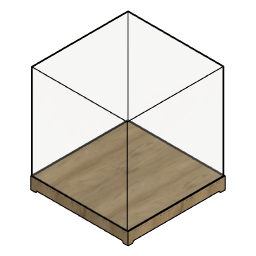
Base_paraiso (Autodesk Fusion 360 design; units mm, degrees)
Autodesk Fusion 360 part; units mm, degrees
sketch "Sketch3" plane through (0, 0, 0) normal (0, 0, 1) x (1, 0, 0)
  line L0 (-400, -400) -> (400, -400)
  line L1 (400, -400) -> (400, 400)
  line L2 (400, 400) -> (-400, 400)
  line L3 (-400, 400) -> (-400, -400)
  line L4 (382, -382) -> (382, 382)
  line L5 (382, 382) -> (-382, 382)
  line L6 (-382, 382) -> (-382, -382)
  line L7 (-382, -382) -> (382, -382)
  line L8 (-400, 400) -> (-382, 382)
  line L9 (382, -382) -> (400, -400)
  line L10 (-400, -400) -> (-382, -382)
  line L11 (382, 382) -> (400, 400)
  line L12 (-400, -400) -> (-382, -382) construction
  line L13 (382, 382) -> (400, 400) construction
  line L14 (400, -400) -> (382, -382) construction
  line L15 (-382, 382) -> (-400, 400) construction
  dimension "d11" = 800
  dimension "d12" = 800
  dimension "d13" = -18
  constraint horizontal L0
  constraint perpendicular L0 L1
  constraint parallel L0 L2
  constraint parallel L1 L3
  constraint coincident origin L12
  constraint coincident origin L14
  constraint parallel L8 L14
  constraint collinear L8 L9
  constraint collinear L10 L11
  constraint collinear L12 L13
  constraint collinear L14 L15
  measures "d11" distance of L1.end L2.end
  measures "d12" distance of L0.end L1.end
extrude "Extrude3" add sketch "Sketch3" along normal blind 100 contours L3 L6 L8 L10 | L1 L4 L9 L11 makes body 1 at (-400, 133.3333, 66.6667) makes body 2 at (400, -133.3333, 66.6667)
extrude "Extrude4" add sketch "Sketch3" along normal blind 100 separate body contours L0 L7 L9 L10 | L2 L5 L8 L11 makes body 3 at (-133.3333, -400, 66.6667) makes body 4 at (133.3333, 400, 66.6667)
sketch "Sketch4" plane through (0, -400, 0) normal (0, -1, 0) x (1, 0, 0)
  line L0 (-400, 0) -> (400, 0)
  line L1 (400, 0) -> (400, 100)
  line L2 (400, 100) -> (-400, 100)
  line L3 (-400, 100) -> (-400, 0)
  line L4 (-350, 0) -> (0, 0)
  line L5 (-350, 15) -> (0, 15)
  line L6 (-350, 0) -> (-365, 0)
  arc A0 (-350, 15) -> (-365, 0) centre (-350, 0) ccw
  spline S0 degree 5 poles (0, 0) (0, 7.6752) (0, 23.0256) (0, 46.0513) (0, 76.7521) (0, 115.1282) (0, 145.829) (0, 168.8546) (0, 184.2051) (0, 191.8803) knots 0 0 0 0 0 0 0.2 0.4 0.6 0.8 1 1 1 1 1 1 construction
  line L7 (0, 1.75) -> (0, 22.5) construction
  line L8 (350, 0) -> (0, 0)
  line L9 (350, 0) -> (365, 0)
  arc A1 (365, 0) -> (350, 15) centre (350, 0) ccw
  line L10 (350, 15) -> (0, 15)
  point P0 (-400, 0)
  dimension "d18" = -15
  dimension "d19" = 50
  constraint coincident L0 L4.start
  constraint coincident L4.end S0.start
  constraint perpendicular L3 L4
  constraint coincident L4.start L6.start
  constraint tangent L5 A0
  constraint coincident L0 L6.end
  constraint symmetric L4.start L7 L8.start
  constraint symmetric L4.end L7 S0.start
  constraint symmetric L5.start L7 A1.end
  constraint symmetric L5.end L7 L10.end
  constraint symmetric L6.end L7 L9.end
  constraint symmetric A0 L7 A1
  measures "d19" distance of L4.start P0
ref_plane "WorkPlane1" through (0, -400, 50) normal (0, -1, 0) x (1, 0, 0)
sketch "Sketch6" plane through (0, 0, 100) normal (0, 0, 1) x (-1, 0, 0)
  line L0 (400, 400) -> (-400, 400)
  line L1 (-400, 400) -> (-382, 382)
  line L2 (-382, 382) -> (382, 382)
  line L3 (382, 382) -> (400, 400)
  line L4 (394, 394) -> (-394, 394)
  line L5 (-394, 394) -> (-394, -394)
  line L6 (-394, -394) -> (394, -394)
  line L7 (394, -394) -> (394, 394)
  line L8 (394, 394) -> (-394, -394) construction
  line L9 (-394, 394) -> (394, -394) construction
  dimension "d38" = 12
  constraint horizontal L4
  constraint perpendicular L4 L5
  constraint parallel L4 L6
  constraint parallel L5 L7
  constraint coincident L8 origin
  constraint coincident L9 origin
  measures "d38" distance of L2 L4
extrude "Extrude8" cut sketch "Sketch6" against normal blind 20 contours L1 L2 L3 L5 L6 L7 | L1 L2 L3 L4 bodies 1 2 3 4
sketch "Sketch11" plane through (0, -400, 0) normal (0, -1, 0) x (1, 0, 0)
  line L0 (0, 0) -> (0, 171.862) construction
  line L1 (-360, 0) -> (-360, -0.0001)
  line L2 (-345, 15) -> (0, 15)
  arc A0 (-345, 15) -> (-360, -0.0001) centre (-345, 0) ccw
  line L3 (-360, 0) -> (0, 0)
  line L4 (345, 15) -> (0, 15)
  line L5 (360, 0) -> (0, 0)
  arc A1 (360, -0.0001) -> (345, 15) centre (345, 0) ccw
  point P0 (-360.0001, 15)
  point P1 (-400, 0)
  dimension "d67" = 15
  dimension "d68" = 40
  dimension "d69" = 15
  constraint coincident L0.start L3.end
  constraint vertical L0
  constraint coincident L0 L2.end
  constraint perpendicular L0 L2
  constraint coincident P0 L1
  constraint coincident P0 L2
  constraint tangent L1 A0
  constraint tangent L2 A0
  constraint perpendicular L0 L3
  constraint symmetric L0 L1.start L5.start
  constraint symmetric L0 L2.end L4.end
  constraint symmetric L0 L1.end A1.start
  constraint symmetric L0 L2.start L4.start
  constraint symmetric L0 A0 A1
  constraint symmetric L0 L3.end L5.end
  measures "d67" distance of L1.start P0
  measures "d68" distance of L1.start P1
  measures "d69" radius of A0
extrude "Extrude12" cut sketch "Sketch11" against normal blind 840 bodies 3 4
sketch "Sketch12" plane through (-400, 0, 0) normal (-1, 0, 0) x (0, -1, 0)
  line L0 (-400, 0) -> (400, 0)
  line L1 (400, 0) -> (400, 100)
  line L2 (400, 100) -> (-400, 100)
  line L3 (-400, 100) -> (-400, 0)
  line L4 (0, 0) -> (0, 212.8854) construction
  line L5 (-360, 0) -> (-360, 0.5)
  line L6 (-345.5, 15) -> (0, 15)
  arc A0 (-345.5, 15) -> (-360, 0.5) centre (-345.5, 0.5) ccw
  line L7 (-360, 0) -> (0, 0)
  line L8 (345.5, 15) -> (0, 15)
  arc A1 (360, 0.5) -> (345.5, 15) centre (345.5, 0.5) ccw
  line L9 (360, 0) -> (0, 0)
  line L10 (360, 0.5) -> (360, 0)
  point P0 (-360, 15)
  dimension "d76" = 40
  dimension "d77" = 15
  dimension "d78" = 14.5
  constraint coincident L4.start L7.end
  constraint perpendicular L0 L4
  constraint coincident L0 L5.start
  constraint perpendicular L0 L5
  constraint coincident L4 L6.end
  constraint perpendicular L4 L6
  constraint coincident P0 L5
  constraint coincident P0 L6
  constraint tangent L5 A0
  constraint tangent L6 A0
  constraint symmetric L4 L5.start L9.start
  constraint symmetric L4 L6.end L8.end
  constraint symmetric L4 L5.end A1.start
  constraint symmetric L4 L6.start L8.start
  constraint symmetric L4 A0 A1
  constraint symmetric L4 L7.end L9.end
  measures "d76" distance of L0.start L5.start
  measures "d77" distance of L5.start P0
  measures "d78" radius of A0
extrude "Extrude13" cut sketch "Sketch12" against normal blind 950 contours L0 L5 L6 A0 L7 L8 A1 L9 L10 bodies 2 1
sketch "Sketch13" plane through (0, 0, 100) normal (0, 0, 1) x (-1, 0, 0)
  line L0 (394, -394) -> (-394, -394)
  line L1 (-394, -394) -> (-400, -400)
  line L2 (-400, -400) -> (400, -400)
  line L3 (400, -400) -> (394, -394)
  line L4 (391, -391) -> (-391, -391)
  line L5 (-391, -391) -> (-391, 391)
  line L6 (-391, 391) -> (391, 391)
  line L7 (391, 391) -> (391, -391)
  line L8 (391, -391) -> (-391, 391) construction
  line L9 (-391, -391) -> (391, 391) construction
  dimension "d81" = 3
  constraint horizontal L4
  constraint perpendicular L4 L5
  constraint parallel L4 L6
  constraint parallel L5 L7
  constraint coincident L8 origin
  constraint coincident L9 origin
  measures "d81" distance of L0 L4
extrude "Extrude14" add sketch "Sketch13" along normal blind 19 from surface at -20 separate body contours L4 L5 L6 L7 makes body 5
sketch "Sketch14" plane through (0, -400, 0) normal (0, -1, 0) x (1, 0, 0)
  arc A0 (360, 0) -> (345, 15) centre (345, 0) ccw
  line L0 (360, 0) -> (400, 0)
  line L1 (400, 0) -> (400, 100)
  line L2 (400, 100) -> (-400, 100)
  line L3 (-400, 100) -> (-400, 0)
  line L4 (-400, 0) -> (-360, 0)
  arc A1 (-345, 15) -> (-360, 0) centre (-345, 0) ccw
  line L5 (-345, 15) -> (345, 15)
  line L6 (-393.7875, 80.4321) -> (394.0376, 80.4321)
  line L7 (394.0376, 80.4321) -> (394.0376, 880.4321)
  line L8 (394.0376, 880.4321) -> (-393.7875, 880.4321)
  line L9 (-393.7875, 880.4321) -> (-393.7875, 80.4321)
  dimension "d85" = 800
  constraint horizontal L6
  constraint vertical L7
  constraint horizontal L8
  constraint vertical L9
  measures "d85" distance of L6.start L8.end
extrude "Extrude15" add sketch "Sketch14" against normal blind 794 separate body contours L2 L7 L8 L9 makes body 6
shell "Shell1" thickness 3 removed faces 1 at (131.4293, -135.3333, 100) on bodies 6
